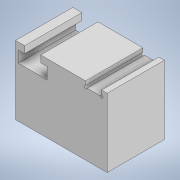
# Autodesk Inventor part: PiesaSuportCanale
Saved by Autodesk Inventor 2021 (Build 250183000, 183)
## iProperties
Created: 2021-03-10
Part Number: PiesaSuportCanale
Material: Generic
Document SubType Name: Modeling
Designer: Crist
Density: 1 g/cm^3
Appearance: Default
Author: Crist
Autodesk Inventor part; units mm, degrees
ref_plane "YZ Plane" through (0, 0, 0) normal (1, 0, 0) x (0, 1, 0)
ref_plane "XZ Plane" through (0, 0, 0) normal (0, 1, 0) x (-1, 0, 0)
ref_plane "XY Plane" through (0, 0, 0) normal (0, 0, 1) x (1, 0, 0)
sketch "Sketch1" plane through (0, 0, 0) normal (0, 0, 1) x (1, 0, 0)
  line L0 (-36.9152, 36.2425) -> (43.0848, 36.2425)
  line L1 (43.0848, 36.2425) -> (43.0848, -23.7575)
  line L2 (43.0848, -23.7575) -> (-36.9152, -23.7575)
  line L3 (-36.9152, -23.7575) -> (-36.9152, 36.2425)
  point P0 (0, 0)
  dimension "d0" = 80
  dimension "d1" = 60
  constraints: 8 end point, 2 parallel, 1 horizontal, 1 perpendicular
  measures "d0" distance of L0.start L0.end
  measures "d1" distance of L2.end L0.start
extrude "Extrusion1" add sketch "Sketch1" along normal blind 50
sketch "Sketch2" plane through (0, 0, 50) normal (0, 0, 1) x (1, 0, 0)
  line L0 (-34.4619, 20.2567) -> (-34.4619, 30.2567)
  line L1 (-34.4619, 30.2567) -> (-28.9619, 30.2567)
  line L2 (-28.9619, 30.2567) -> (-28.9619, 39.2567)
  line L3 (-28.9619, 39.2567) -> (-14.9619, 39.2567)
  line L4 (-14.9619, 39.2567) -> (-14.9619, 30.2567)
  line L5 (-14.9619, 30.2567) -> (-9.4619, 30.2567)
  line L6 (-9.4619, 30.2567) -> (-9.4619, 20.2567)
  line L7 (-9.4619, 20.2567) -> (-34.4619, 20.2567)
  point P0 (0, 0)
  point P1 (-21.9619, 39.2567)
  dimension "d4" = 14
  dimension "d5" = 9
  dimension "d6" = 10
  dimension "d7" = 12.5
  dimension "d8" = 25
  dimension "d9" = 7
  constraints: 16 end point, 6 perpendicular, 2 point on line, 1 midpoint, 1 vertical
  measures "d4" distance of L2.end L3.end
  measures "d5" distance of L1.end L2.end
  measures "d6" distance of L0.start L0.end
  measures "d7" distance from line of L0 point (-21.962, 39.257)
  measures "d8" distance of L6.end L0.start
  measures "d9" distance of L2.end point (-21.962, 39.257)
extrude "Extrusion2" cut sketch "Sketch2" against normal blind 50
sketch "Sketch5" plane through (0, 0, 50) normal (0, 0, 1) x (1, 0, 0)
  line L0 (31.2523, 36.3999) -> (38.2523, 36.3999)
  line L1 (38.2523, 36.3999) -> (38.2523, 32.8141)
  line L2 (38.2523, 32.8141) -> (39.6665, 31.3999)
  line L3 (39.6665, 31.3999) -> (38.2523, 29.9857)
  line L4 (38.2523, 29.9857) -> (36.8381, 31.3999)
  line L5 (36.8381, 31.3999) -> (31.2523, 31.3999)
  line L6 (31.2523, 36.3999) -> (31.2523, 31.3999) construction
  line L7 (31.2523, 36.3999) -> (24.2523, 36.3999)
  line L8 (24.2523, 36.3999) -> (24.2523, 32.8141)
  line L9 (24.2523, 32.8141) -> (22.8381, 31.3999)
  line L10 (22.8381, 31.3999) -> (24.2523, 29.9857)
  line L11 (24.2523, 29.9857) -> (25.6665, 31.3999)
  line L12 (25.6665, 31.3999) -> (31.2523, 31.3999)
  point P0 (0, 0)
  dimension "d27" = 7
  dimension "d28" = 2
  dimension "d29" = 2
  dimension "d30" = 135
  dimension "d31" = 90
  dimension "d32" = 5
  dimension "d33" = 2
  constraints: 26 end point, 5 symmetric about line, 2 perpendicular, 1 coincident, 1 horizontal, 1 parallel, 1 vertical
  measures "d27" distance of L0.start L0.end
  measures "d28" distance of L1.end L2.end
  measures "d29" distance of L2.end L3.end
  measures "d30" angle of L4 L5
  measures "d31" angle of L3 L2
  measures "d32" distance from line of L5 L0.start
  measures "d33" distance of L3.end L4.end
extrude "Extrusion3" cut sketch "Sketch5" against normal blind 50
body "Solid1"
